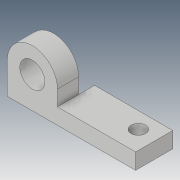
# Autodesk Inventor part: axleMount
Saved by Autodesk Inventor 2018 (Build 220112000, 112)
## iProperties
Created: 2020-01-20
Part Number: axleMount
Material: Generic
Document SubType Name: Modeling
Designer: anirudh
Density: 1 g/cm^3
Appearance: Default
Author: anirudh
Autodesk Inventor part; units mm, degrees
ref_plane "YZ Plane" through (0, 0, 0) normal (1, 0, 0) x (0, 1, 0)
ref_plane "XZ Plane" through (0, 0, 0) normal (0, 1, 0) x (-1, 0, 0)
ref_plane "XY Plane" through (0, 0, 0) normal (0, 0, 1) x (1, 0, 0)
sketch "Sketch1" plane through (0, 0, 0) normal (0, 0, 1) x (1, 0, 0)
  arc A0 (6, 0) -> (-6, 0) centre (0, 0) ccw
  circle A1 centre (0, 0) radius 3
  line L0 (-6, 0) -> (-6, -6)
  line L1 (-6, -6) -> (0, -6)
  line L2 (0, -6) -> (6, -6)
  line L3 (6, -6) -> (18.7, -6)
  line L4 (18.7, -6) -> (18.7, 0)
  line L5 (18.7, 0) -> (6, 0)
  dimension "d4" = 12
  dimension "d5" = 6
  constraints: 12 end point, 2 centre point, 2 perpendicular, 2 point on circle, 2 vertical, 1 coincident, 1 horizontal, 1 point on line, 1 tangent
  measures "d4" diameter of A0
  measures "d5" diameter of A1
extrude "Extrusion1" add sketch "Sketch1" along normal blind 5.08
sketch "Sketch3" plane through (-6, -6, 0) normal (0, -1, 0) x (1, 0, 0)
  line L0 (24.7, 0) -> (24.7, 5.08) projected
  line L1 (0, 5.08) -> (24.7, 5.08) projected
  line L2 (24.7, 0) -> (0, 0)
  line L3 (0, 0) -> (0, 5.08)
  line L4 (0, 5.08) -> (24.7, 5.08)
  line L5 (24.7, 5.08) -> (24.7, 0)
  point P0 (6, 0)
  constraints: 8 end point, 2 parallel, 1 horizontal, 1 perpendicular
extrude "Extrusion3" add sketch "Sketch3" along normal blind 1.4986
sketch "Sketch4" plane through (6, 0, 0) normal (0, 1, 0) x (1, 0, 0)
  line L0 (12.7, 0) -> (12.7, -5.08) projected
  line L1 (12.7, -5.08) -> (0, -5.08)
  line L2 (0, -5.08) -> (0, 0)
  line L3 (0, 0) -> (12.7, 0)
  line L4 (12.7, 0) -> (12.7, -5.08)
  point P0 (-6, 0)
  constraints: 8 end point, 2 parallel, 1 horizontal, 1 perpendicular
extrude "Extrusion4" cut sketch "Sketch4" against normal blind 3.683
sketch "Sketch5" plane through (18.7, -7.4986, 5.08) normal (1, 0, 0) x (0, 0, -1)
  line L0 (0, 3.8156) -> (0, 0) projected
  line L1 (5.08, 0) -> (0, 0) projected
  line L2 (0, 3.8156) -> (5.08, 3.8156)
  line L3 (5.08, 3.8156) -> (5.08, 0)
  line L4 (5.08, 0) -> (0, 0)
  line L5 (0, 0) -> (0, 3.8156)
  point P0 (5.08, 7.4986)
  constraints: 8 end point, 2 parallel, 1 horizontal, 1 perpendicular
extrude "Extrusion5" add sketch "Sketch5" along normal blind 6
sketch "Sketch6" plane through (6, -3.683, 0) normal (0, 1, 0) x (1, 0, 0)
  line L0 (0, 0) -> (-12, 0) projected
  line L1 (0, 0) -> (18.7, 0)
  line L2 (18.7, 0) -> (18.7, 3.81)
  line L3 (18.7, 3.81) -> (0, 3.81)
  line L4 (0, 3.81) -> (0, 0)
  point P0 (-6, 0)
  dimension "d19" = 3.81
  constraints: 8 end point, 2 parallel, 1 horizontal, 1 perpendicular
  measures "d19" distance of L2.end L1.end
extrude "Extrusion6" add sketch "Sketch6" against normal blind 3.81
sketch "Sketch7" plane through (6, -3.683, 0) normal (0, 1, 0) x (1, 0, 0)
  line L0 (18.7, -5.08) -> (18.7, 3.81) projected
  line L1 (18.7, -5.08) -> (0, -5.08) projected
  circle A0 centre (14.3566, -0.0762) radius 1.75
  point P0 (-6, 0)
  dimension "d25" = 3.5
  constraints: 1 centre point
  measures "d25" diameter of A0
extrude "Extrusion7" cut sketch "Sketch7" against normal blind 5.3975
body "Solid1"
